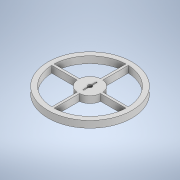
# Autodesk Inventor part: Pot Disk
Saved by Autodesk Inventor 2022 (Build 260153000, 153)
## iProperties
Created: 2023-03-08
Part Number: Pot Disk
Material: Generic
Document SubType Name: Modeling
Designer: Jacki
Density: 1 g/cm^3
Appearance: Default
Author: Jacki
Autodesk Inventor part; units mm, degrees
ref_plane "YZ Plane" through (0, 0, 0) normal (1, 0, 0) x (0, 1, 0)
ref_plane "XZ Plane" through (0, 0, 0) normal (0, 1, 0) x (-1, 0, 0)
ref_plane "XY Plane" through (0, 0, 0) normal (0, 0, 1) x (1, 0, 0)
sketch "Sketch1" plane through (0, 0, 0) normal (0, 1, 0) x (-1, 0, 0)
  circle A0 centre (0, 0) radius 62.2958
  line L0 (-0.7, -10) -> (0.7, -10)
  line L1 (0.6998, 10) -> (-0.7, 10)
  line L2 (0.7, -10) -> (0.7, -2.8135)
  line L3 (0.6998, 2.8135) -> (0.6998, 10)
  line L4 (-0.7, 10) -> (-0.7, 2.8142)
  line L5 (-0.7, -2.8142) -> (-0.7, -10)
  arc A1 (-0.7, 2.8142) -> (-0.7, -2.8142) centre (0, 0) ccw
  arc A2 (0.7, -2.8135) -> (0.6998, 2.8135) centre (0, 0) ccw
  dimension "d0" = 124.5916
  dimension "d2" = 1.4
  dimension "d6" = 20
  dimension "d7" = 10
  constraints: 12 end point, 5 parallel, 4 point on circle, 3 centre point, 2 coincident, 2 perpendicular, 2 vertical
  measures "d0" diameter of A0
  measures "d2" distance of L0.end L0.start
  measures "d6" distance between parallel lines of L0 L1
  measures "d7" distance from line of L1 point (0, 0)
extrude "Extrusion1" add sketch "Sketch1" along normal blind 10
sketch "Sketch4" plane through (0, 0, 0) normal (0, -1, 0) x (1, 0, 0)
  point P0 (0, 0)
sketch "Sketch6" plane through (0, 0, 0) normal (0, -1, 0) x (1, 0, 0)
  circle A0 centre (0, 0) radius 17.5
  line L0 (70.933, -2.5) -> (70.933, 2.5)
  line L1 (-76.7315, 1.75) -> (-76.7315, -1.75)
  arc A1 (-0.6998, 2.8135) -> (-0.7, -2.8135) centre (0, 0) ccw projected
  arc A2 (0.7, -2.8142) -> (0.7, 2.8142) centre (0, 0) ccw projected
  circle A3 centre (0, 0) radius 55
  line L2 (2.5, 115.1017) -> (-2.5, 115.1017)
  line L3 (-2.5, -115.1017) -> (2.5, -115.1017)
  line L4 (0.7, 10) -> (-0.6998, 10) projected
  circle A4 centre (0, 0) radius 62.2958
  line L5 (-76.7315, -1.75) -> (-17.4123, -1.75)
  line L6 (-17.4123, 1.75) -> (-76.7315, 1.75)
  line L7 (-1.4682, 2.5) -> (-1.4697, 2.5)
  line L8 (-1.75, -17.4123) -> (-1.75, -76.7315)
  line L9 (1.75, -76.7315) -> (1.75, -17.4123)
  line L10 (17.4123, -1.75) -> (76.7315, -1.75)
  line L11 (76.7315, 1.75) -> (17.4123, 1.75)
  line L12 (1.75, 17.4123) -> (1.75, 76.7315)
  line L13 (-1.75, 76.7315) -> (-1.75, 17.4123)
  point P0 (-2.8993, 0)
  point P1 (-2.5, 17.3205)
  point P2 (-2.5, -17.3205)
  point P3 (2.5, -17.3205)
  point P4 (17.3205, -2.5)
  point P5 (17.3205, 2.5)
  point P6 (2.5, 17.3205)
  point P7 (-54.9722, 1.75)
  point P8 (-54.9722, -1.75)
  point P9 (54.9722, -1.75)
  point P10 (1.75, -54.9722)
  point P11 (1.75, 54.9722)
  point P12 (54.9722, 1.75)
  point P13 (-1.75, 54.9722)
  point P14 (-1.75, -54.9722)
  dimension "d16" = 35
  dimension "d18" = 110
  dimension "d19" = 5
  dimension "d22" = 1.75
  dimension "d23" = 3.5
  dimension "d26" = 360
  constraints: 26 end point, 4 parallel, 3 coincident, 3 point on circle, 2 centre point, 2 perpendicular, 1 vertical, 35 other
  measures "d18" diameter of A3
  measures "d19" distance of L2.end L2.start
  measures "d22" distance from line of point (0, 0) L6
  measures "d23" distance between parallel lines of L6 L5
extrude "Extrusion2" cut sketch "Sketch6" against normal blind 10 contours A0 L12 A3 L11 | L10 A3 L9 A0 | A0 L6 A3 L13 | L8 A3 L5 A0
body "Solid1"
